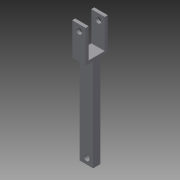
# Autodesk Inventor part: UpperLeg_v2
Saved by Autodesk Inventor 2013 (Build 170138000, 138)
## iProperties
Created: 2012-11-28
Part Number: UpperLeg_v2
Material: Generic
Document SubType Name: Modeling
Designer: Joe
Density: 1 g/cm^3
Author: Joe
Autodesk Inventor part; units mm, degrees
ref_plane "YZ Plane" through (0, 0, 0) normal (1, 0, 0) x (0, 1, 0)
ref_plane "XZ Plane" through (0, 0, 0) normal (0, 1, 0) x (-1, 0, 0)
ref_plane "XY Plane" through (0, 0, 0) normal (0, 0, 1) x (1, 0, 0)
sketch "Sketch1" plane through (0, 0, 0) normal (1, 0, 0) x (0, 1, 0)
  circle A0 centre (0, 0) radius 10
  circle A1 centre (-379, 0) radius 10
  line L0 (0, 0) -> (-379, 0) construction
  line L1 (20, 22.5) -> (-399, 22.5)
  line L2 (-399, 22.5) -> (-399, -22.5)
  line L3 (-399, -22.5) -> (20, -22.5)
  line L4 (20, -22.5) -> (20, 22.5)
  line L5 (20, 0) -> (-399, 0) construction
  dimension "d0" = 20
  dimension "d2" = 20
  dimension "d3" = 379
  dimension "d4" = 45
  dimension "d5" = 20
  constraints: 12 end point, 2 centre point, 2 horizontal, 2 midpoint, 2 parallel, 1 coincident, 1 collinear, 1 equal radius, 1 perpendicular
  measures "d0" distance from line of L4 L0.start
  measures "d2" distance from line of L2 L0.end
  measures "d3" distance of L0.start L0.end
  measures "d4" distance of L3.end L1.start
  measures "d5" diameter of A0
extrude "Extrusion1" add sketch "Sketch1" along normal mid plane 24
sketch "Sketch2" plane through (12, 0, 0) normal (1, 0, 0) x (0, 0, -1)
  circle A0 centre (0, 0) radius 10 projected
  line L0 (22.5, -399) -> (22.5, 20) projected
  line L1 (22.5, 20) -> (-22.5, 20) projected
  line L2 (-22.5, 20) -> (22.5, 20)
  line L3 (22.5, 20) -> (22.5, -89)
  line L4 (22.5, -89) -> (-22.5, -89)
  line L5 (-22.5, -89) -> (-22.5, 20)
  circle A1 centre (0, 0) radius 10
  dimension "d8" = 109
  constraints: 8 end point, 2 parallel, 1 centre point, 1 coincident, 1 concentric, 1 horizontal, 1 perpendicular, 1 point on line
  measures "d8" distance of L4.end L1.end
extrude "Extrusion2" add sketch "Sketch2" along normal blind 25
mirror "Mirror1" about plane through (0, 0, 0) normal (1, 0, 0) of "Extrusion2"
sketch "Sketch3" plane through (-12, -399, 22.5) normal (0, 0, 1) x (1, 0, 0)
  line L0 (49, 419) -> (-25, 419) projected
  line L1 (-15, 419) -> (39, 419)
  line L2 (39, 419) -> (39, 320)
  line L3 (39, 320) -> (-15, 320)
  line L4 (-15, 320) -> (-15, 419)
  line L5 (12, 419) -> (12, 320) construction
  point P0 (12, 399)
  dimension "d11" = 99
  dimension "d13" = 54
  constraints: 10 end point, 2 midpoint, 2 parallel, 2 point on line, 1 horizontal, 1 perpendicular
  measures "d11" distance of L3.end L1.start
  measures "d13" distance of L2.end L3.end
extrude "Extrusion3" cut sketch "Sketch3" against normal through all
move or copy body "Move Body1" bodies to move or copy 1 copy no rotation origin (0, 0, 0) rotation axis (1, 0, 0) rotation angle 90
move or copy body "Move Body2" bodies to move or copy 1 copy no rotation origin (0, 0, 0) rotation axis (0, 0, 1) rotation angle 90
body "Solid1"
